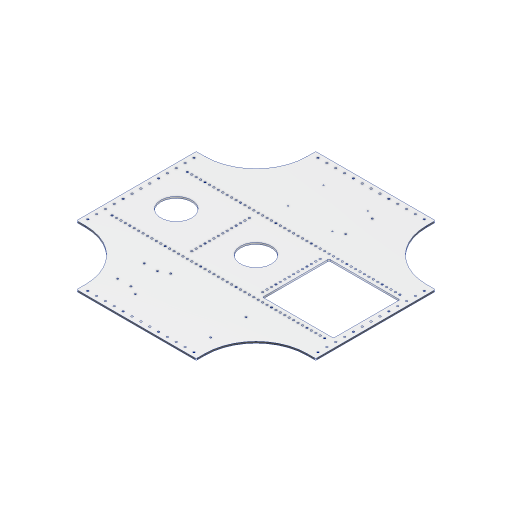
# Autodesk Inventor part: 27in_2_125 belly pan_Green
Saved by Autodesk Inventor 2023 (Build 270158000, 158)
## iProperties
Created: 2023-10-28
Part Number: 27in_2_125 belly pan_Green
Material: Aluminum 6061
Document SubType Name: Modeling
Designer: jackc
Density: 2.7 g/cm^3
Appearance: Aluminum - Flat
Author: jackc
Autodesk Inventor part; units mm, degrees
ref_plane "YZ Plane" through (0, 0, 0) normal (1, 0, 0) x (0, 1, 0)
ref_plane "XZ Plane" through (0, 0, 0) normal (0, 1, 0) x (-1, 0, 0)
ref_plane "XY Plane" through (0, 0, 0) normal (0, 0, 1) x (1, 0, 0)
sketch "Sketch1" plane through (0, 0, 0) normal (0, 1, 0) x (-1, 0, 0)
  line L0 (685.8, 0) -> (685.8, -342.9)
  line L1 (0, 0) -> (0, -342.9)
  line L2 (514.35, -514.35) -> (171.45, -514.35)
  line L3 (514.35, 171.45) -> (171.45, 171.45)
  line L4 (685.8, 0) -> (685.8, 171.45) construction
  line L5 (685.8, 171.45) -> (514.35, 171.45) construction
  line L6 (685.8, -342.9) -> (685.8, -514.35) construction
  line L7 (685.8, -514.35) -> (514.35, -514.35) construction
  line L8 (0, -342.9) -> (0, -514.35) construction
  line L9 (0, -514.35) -> (171.45, -514.35) construction
  line L10 (685.8, 0) -> (660.4, 0)
  line L11 (514.35, 171.45) -> (514.35, 146.05)
  line L12 (171.45, 171.45) -> (171.45, 146.05)
  line L13 (0, 0) -> (25.4, 0)
  line L14 (0, -342.9) -> (25.4, -342.9)
  line L15 (171.45, -514.35) -> (171.45, -488.95)
  line L16 (685.8, -342.9) -> (660.4, -342.9)
  line L17 (514.35, -514.35) -> (514.35, -488.95)
  arc A0 (514.35, 146.05) -> (660.4, 0) centre (660.4, 146.05) ccw
  arc A1 (25.4, 0) -> (171.45, 146.05) centre (25.4, 146.05) ccw
  arc A2 (171.45, -488.95) -> (25.4, -342.9) centre (25.4, -488.95) ccw
  arc A3 (660.4, -342.9) -> (514.35, -488.95) centre (660.4, -488.95) ccw
  dimension "d2" = 685.8
  dimension "d14" = 171.45
  dimension "d15" = 25.4
  dimension "d16" = 25.4
  dimension "d17" = 25.4
  dimension "d18" = 25.4
  dimension "d19" = 25.4
  dimension "d21" = 25.4
  dimension "d22" = 25.4
  constraints: 36 end point, 11 equal length, 8 point on circle, 8 vertical, 6 perpendicular, 4 centre point, 4 horizontal, 2 horizontal alignment, 1 coincident, 1 equal radius
  measures "d2" distance of L6.end L4.end
  measures "d14" distance of L0.start L4.end
  measures "d15" distance of L0.start L10.end
  measures "d16" distance of L1.start L13.end
  measures "d17" distance of L1.end L14.end
  measures "d18" distance of L2.end L15.end
  measures "d19" horizontal distance of A0.centre L4.end
  measures "d21" horizontal distance of L8.end A2.centre
  measures "d22" horizontal distance of A1.centre L8.end
extrude "Extrusion1" add sketch "Sketch1" along normal blind 4.7752
sketch "Sketch2" plane through (0, 0, 0) normal (0, 1, 0) x (1, 0, 0)
  line L0 (-685.8, 342.9) -> (-685.8, 0) projected
  line L1 (-685.8, 50.8) -> (0, 50.8) construction
  line L2 (0, 342.9) -> (0, 0) projected
  line L3 (-0.228, 76.2) -> (-685.8, 76.2) construction
  line L4 (-685.8, 266.7) -> (0, 266.7) construction
  line L5 (0, 292.1) -> (-685.8, 292.1) construction
  line L6 (-685.8, 0) -> (-685.8, 342.9) projected
  arc A0 (-514.35, -146.05) -> (-660.4, 0) centre (-660.4, -146.05) ccw construction
  arc A1 (-660.4, 342.9) -> (-514.35, 488.95) centre (-660.4, 488.95) ccw construction
  line L7 (-660.4, 0) -> (-660.4, 342.9) construction
  line L8 (-469.9, 76.2) -> (-469.9, 266.7) construction
  circle A2 centre (-571.5, 171.45) radius 44.45
  line L9 (-444.5, 76.2) -> (-444.5, 266.7) construction
  line L10 (-342.9, 76.2) -> (-342.9, 266.7) construction
  line L11 (-241.3, 76.2) -> (-241.3, 266.7) construction
  circle A3 centre (-444.5, 88.9) radius 2.8067
  circle A4 centre (-241.3, 88.9) radius 2.8067
  circle A5 centre (-444.5, 114.3) radius 2.8067
  circle A6 centre (-241.3, 114.3) radius 2.8067
  circle A7 centre (-444.5, 139.7) radius 2.8067
  circle A8 centre (-241.3, 139.7) radius 2.8067
  circle A9 centre (-444.5, 165.1) radius 2.8067
  circle A10 centre (-241.3, 165.1) radius 2.8067
  circle A11 centre (-444.5, 190.5) radius 2.8067
  circle A12 centre (-241.3, 190.5) radius 2.8067
  circle A13 centre (-444.5, 215.9) radius 2.8067
  circle A14 centre (-241.3, 215.9) radius 2.8067
  circle A15 centre (-444.5, 241.3) radius 2.8067
  circle A16 centre (-241.3, 241.3) radius 2.8067
  circle A17 centre (-342.9, 171.45) radius 44.45
  line L12 (-228.6, 76.2) -> (-228.6, 266.7)
  line L13 (-25.4, 76.2) -> (-25.4, 266.7)
  line L14 (-228.6, 266.7) -> (-25.4, 266.7)
  line L15 (-25.4, 76.2) -> (-228.6, 76.2)
  circle A18 centre (-444.5, 254) radius 2.8067
  circle A19 centre (-241.3, 254) radius 2.8067
  circle A20 centre (-444.5, 228.6) radius 2.8067
  circle A21 centre (-241.3, 228.6) radius 2.8067
  circle A22 centre (-444.5, 203.2) radius 2.8067
  circle A23 centre (-241.3, 203.2) radius 2.8067
  circle A24 centre (-444.5, 177.8) radius 2.8067
  circle A25 centre (-241.3, 177.8) radius 2.8067
  circle A26 centre (-444.5, 152.4) radius 2.8067
  circle A27 centre (-241.3, 152.4) radius 2.8067
  circle A28 centre (-444.5, 127) radius 2.8067
  circle A29 centre (-241.3, 127) radius 2.8067
  circle A30 centre (-444.5, 101.6) radius 2.8067
  circle A31 centre (-241.3, 101.6) radius 2.8067
  point P0 (-660.4, 171.45)
  dimension "d2" = 685.8
  dimension "d14" = 171.45
  dimension "d15" = 25.4
  dimension "d16" = 25.4
  dimension "d17" = 25.4
  dimension "d18" = 25.4
  dimension "d19" = 25.4
  dimension "d21" = 25.4
  dimension "d22" = 25.4
  dimension "d23" = 25.4
  dimension "d24" = 25.4
  dimension "d25" = 190.5
  dimension "d26" = 50.8
  dimension "d31" = 190.5
  dimension "d47" = 88.9
  dimension "d48" = 88.9
  dimension "d49" = 342.9
  dimension "d50" = 101.6
  dimension "d51" = 101.6
  dimension "d54" = 25.4
  dimension "d61" = 12.7
  dimension "d62" = 25.4
  dimension "d100" = 5.6134
  dimension "d101" = 12.7
  dimension "d102" = 12.7
  dimension "d105" = 25.4
  constraints: 30 centre point, 26 end point, 22 point on line, 6 perpendicular, 4 equal radius, 3 horizontal alignment, 3 midpoint, 3 parallel, 3 vertical, 2 collinear, 1 horizontal, 48 other
  measures "d23" distance between parallel lines of L1 L3
  measures "d24" distance between parallel lines of L5 L4
  measures "d25" distance between parallel lines of L4 L3
  measures "d26" distance of L0.start L5.end
  measures "d31" distance between parallel lines of L8 L7
  measures "d47" diameter of A2
  measures "d48" distance of A2.centre point (-660.4, 171.45)
  measures "d49" distance between parallel lines of L10 L2
  measures "d50" distance between parallel lines of L9 L10
  measures "d51" distance between parallel lines of L11 L10
  measures "d54" distance of A3.centre A5.centre
  measures "d61" distance between parallel lines of L11 L12
  measures "d62" distance between parallel lines of L13 L2
  measures "d100" diameter of A15
  measures "d101" distance of L9.start A3.centre
  measures "d102" distance from line of A18.centre L4
  measures "d105" distance of A18.centre A20.centre
sketch "Sketch3" plane through (0, 0, 0) normal (0, 1, 0) x (1, 0, 0)
  line L0 (-419.1, -98.425) -> (-203.2, -98.425) construction
  line L1 (-203.2, -98.425) -> (-203.2, 3.175) construction
  line L2 (-203.2, 3.175) -> (-419.1, 3.175) construction
  line L3 (-419.1, 3.175) -> (-419.1, -98.425) construction
  line L4 (-482.6, -85.725) -> (-444.5, -85.725) construction
  line L5 (-444.5, -85.725) -> (-444.5, -9.525) construction
  line L6 (-444.5, -9.525) -> (-482.6, -9.525) construction
  line L7 (-482.6, -9.525) -> (-482.6, -85.725) construction
  line L8 (-171.45, -171.45) -> (-514.35, -171.45) construction
  circle A0 centre (-419.1, -98.425) radius 2.4892
  circle A1 centre (-444.5, -85.725) radius 2.4892
  circle A2 centre (-482.6, -85.725) radius 2.4892
  circle A3 centre (-482.6, -9.525) radius 2.4892
  circle A4 centre (-419.1, 3.175) radius 2.4892
  circle A5 centre (-203.2, 3.175) radius 2.4892
  circle A6 centre (-203.2, -98.425) radius 2.4892
  circle A7 centre (-444.5, -9.525) radius 2.4892
  point P0 (0, 0)
  dimension "d63" = 101.6
  dimension "d64" = 215.9
  dimension "d65" = 76.2
  dimension "d66" = 38.1
  dimension "d67" = 73.025
  dimension "d68" = 85.725
  dimension "d69" = 31.75
  dimension "d70" = 25.4
  dimension "d71" = 4.9784
  constraints: 16 end point, 8 centre point, 8 coincident, 7 equal radius, 4 parallel, 2 horizontal, 2 perpendicular
  measures "d63" distance of L2.end L0.start
  measures "d64" distance of L1.end L2.end
  measures "d65" distance of L4.end L5.end
  measures "d66" distance of L5.end L6.end
  measures "d67" distance between parallel lines of L0 L8
  measures "d68" distance between parallel lines of L8 L4
  measures "d69" distance from line of L8.start L1
  measures "d70" distance between parallel lines of L3 L5
  measures "d71" diameter of A4
sketch "Sketch4" plane through (0, 0, 0) normal (0, 1, 0) x (1, 0, 0)
  circle A0 centre (-12.7, 323.85) radius 2.8067
  line L0 (0, 342.9) -> (0, 0) projected
  line L1 (-25.4, 342.9) -> (0, 342.9) projected
  circle A1 centre (-12.7, 298.45) radius 2.8067
  circle A2 centre (-12.7, 273.05) radius 2.8067
  circle A3 centre (-12.7, 247.65) radius 2.8067
  circle A4 centre (-12.7, 222.25) radius 2.8067
  circle A5 centre (-12.7, 196.85) radius 2.8067
  circle A6 centre (-12.7, 171.45) radius 2.8067
  circle A7 centre (-12.7, 146.05) radius 2.8067
  circle A8 centre (-12.7, 120.65) radius 2.8067
  circle A9 centre (-12.7, 95.25) radius 2.8067
  circle A10 centre (-12.7, 69.85) radius 2.8067
  circle A11 centre (-12.7, 44.45) radius 2.8067
  circle A12 centre (-12.7, 19.05) radius 2.8067
  circle A13 centre (-419.1, 501.65) radius 2.8067
  circle A14 centre (-393.7, 501.65) radius 2.8067
  circle A15 centre (-368.3, 501.65) radius 2.8067
  circle A16 centre (-317.5, 501.65) radius 2.8067
  circle A17 centre (-292.1, 501.65) radius 2.8067
  circle A18 centre (-266.7, 501.65) radius 2.8067
  circle A19 centre (-241.3, 501.65) radius 2.8067
  circle A20 centre (-215.9, 501.65) radius 2.8067
  circle A21 centre (-190.5, 501.65) radius 2.8067
  circle A22 centre (-342.9, 501.65) radius 2.8067
  circle A23 centre (-444.5, 501.65) radius 2.8067
  circle A24 centre (-469.9, 501.65) radius 2.8067
  circle A25 centre (-495.3, 501.65) radius 2.8067
  circle A26 centre (-673.1, 95.25) radius 2.8067
  circle A27 centre (-673.1, 120.65) radius 2.8067
  circle A28 centre (-673.1, 146.05) radius 2.8067
  circle A29 centre (-673.1, 196.85) radius 2.8067
  circle A30 centre (-673.1, 222.25) radius 2.8067
  circle A31 centre (-673.1, 247.65) radius 2.8067
  circle A32 centre (-673.1, 273.05) radius 2.8067
  circle A33 centre (-673.1, 298.45) radius 2.8067
  circle A34 centre (-673.1, 323.85) radius 2.8067
  circle A35 centre (-673.1, 171.45) radius 2.8067
  circle A36 centre (-673.1, 69.85) radius 2.8067
  circle A37 centre (-673.1, 44.45) radius 2.8067
  circle A38 centre (-673.1, 19.05) radius 2.8067
  circle A39 centre (-266.7, -158.75) radius 2.8067
  circle A40 centre (-292.1, -158.75) radius 2.8067
  circle A41 centre (-317.5, -158.75) radius 2.8067
  circle A42 centre (-368.3, -158.75) radius 2.8067
  circle A43 centre (-393.7, -158.75) radius 2.8067
  circle A44 centre (-419.1, -158.75) radius 2.8067
  circle A45 centre (-444.5, -158.75) radius 2.8067
  circle A46 centre (-469.9, -158.75) radius 2.8067
  circle A47 centre (-495.3, -158.75) radius 2.8067
  circle A48 centre (-342.9, -158.75) radius 2.8067
  circle A49 centre (-241.3, -158.75) radius 2.8067
  circle A50 centre (-215.9, -158.75) radius 2.8067
  circle A51 centre (-190.5, -158.75) radius 2.8067
  circle A52 centre (-38.1, 279.4) radius 2.8067
  line L2 (-228.6, 266.7) -> (-25.4, 266.7)
  line L3 (-228.6, 171.45) -> (-25.4, 171.45) construction
  line L4 (-514.35, 514.35) -> (-171.45, 514.35) construction
  line L5 (-241.3, 171.45) -> (-38.1, 171.45) construction
  circle A53 centre (-50.8, 279.4) radius 2.8067
  line L6 (-254, 171.45) -> (-50.8, 171.45) construction
  circle A54 centre (-63.5, 279.4) radius 2.8067
  line L7 (-266.7, 171.45) -> (-63.5, 171.45) construction
  circle A55 centre (-76.2, 279.4) radius 2.8067
  line L8 (-279.4, 171.45) -> (-76.2, 171.45) construction
  circle A56 centre (-88.9, 279.4) radius 2.8067
  line L9 (-292.1, 171.45) -> (-88.9, 171.45) construction
  circle A57 centre (-101.6, 279.4) radius 2.8067
  line L10 (-304.8, 171.45) -> (-101.6, 171.45) construction
  circle A58 centre (-114.3, 279.4) radius 2.8067
  line L11 (-317.5, 171.45) -> (-114.3, 171.45) construction
  circle A59 centre (-127, 279.4) radius 2.8067
  line L12 (-330.2, 171.45) -> (-127, 171.45) construction
  circle A60 centre (-139.7, 279.4) radius 2.8067
  line L13 (-342.9, 171.45) -> (-139.7, 171.45) construction
  circle A61 centre (-152.4, 279.4) radius 2.8067
  line L14 (-355.6, 171.45) -> (-152.4, 171.45) construction
  circle A62 centre (-165.1, 279.4) radius 2.8067
  line L15 (-368.3, 171.45) -> (-165.1, 171.45) construction
  circle A63 centre (-177.8, 279.4) radius 2.8067
  line L16 (-381, 171.45) -> (-177.8, 171.45) construction
  circle A64 centre (-190.5, 279.4) radius 2.8067
  line L17 (-393.7, 171.45) -> (-190.5, 171.45) construction
  circle A65 centre (-203.2, 279.4) radius 2.8067
  line L18 (-406.4, 171.45) -> (-203.2, 171.45) construction
  circle A66 centre (-215.9, 279.4) radius 2.8067
  line L19 (-419.1, 171.45) -> (-215.9, 171.45) construction
  circle A67 centre (-228.6, 279.4) radius 2.8067
  line L20 (-431.8, 171.45) -> (-228.6, 171.45) construction
  circle A68 centre (-241.3, 279.4) radius 2.8067
  line L21 (-444.5, 171.45) -> (-241.3, 171.45) construction
  circle A69 centre (-254, 279.4) radius 2.8067
  line L22 (-457.2, 171.45) -> (-254, 171.45) construction
  circle A70 centre (-266.7, 279.4) radius 2.8067
  line L23 (-469.9, 171.45) -> (-266.7, 171.45) construction
  circle A71 centre (-279.4, 279.4) radius 2.8067
  line L24 (-482.6, 171.45) -> (-279.4, 171.45) construction
  circle A72 centre (-292.1, 279.4) radius 2.8067
  line L25 (-495.3, 171.45) -> (-292.1, 171.45) construction
  circle A73 centre (-304.8, 279.4) radius 2.8067
  line L26 (-508, 171.45) -> (-304.8, 171.45) construction
  circle A74 centre (-317.5, 279.4) radius 2.8067
  line L27 (-520.7, 171.45) -> (-317.5, 171.45) construction
  circle A75 centre (-330.2, 279.4) radius 2.8067
  line L28 (-533.4, 171.45) -> (-330.2, 171.45) construction
  circle A76 centre (-342.9, 279.4) radius 2.8067
  line L29 (-546.1, 171.45) -> (-342.9, 171.45) construction
  circle A77 centre (-355.6, 279.4) radius 2.8067
  line L30 (-558.8, 171.45) -> (-355.6, 171.45) construction
  circle A78 centre (-368.3, 279.4) radius 2.8067
  line L31 (-571.5, 171.45) -> (-368.3, 171.45) construction
  circle A79 centre (-381, 279.4) radius 2.8067
  line L32 (-584.2, 171.45) -> (-381, 171.45) construction
  circle A80 centre (-393.7, 279.4) radius 2.8067
  line L33 (-596.9, 171.45) -> (-393.7, 171.45) construction
  circle A81 centre (-406.4, 279.4) radius 2.8067
  line L34 (-609.6, 171.45) -> (-406.4, 171.45) construction
  circle A82 centre (-419.1, 279.4) radius 2.8067
  line L35 (-622.3, 171.45) -> (-419.1, 171.45) construction
  circle A83 centre (-431.8, 279.4) radius 2.8067
  line L36 (-635, 171.45) -> (-431.8, 171.45) construction
  circle A84 centre (-444.5, 279.4) radius 2.8067
  line L37 (-647.7, 171.45) -> (-444.5, 171.45) construction
  circle A85 centre (-457.2, 279.4) radius 2.8067
  line L38 (-660.4, 171.45) -> (-457.2, 171.45) construction
  circle A86 centre (-469.9, 279.4) radius 2.8067
  line L39 (-673.1, 171.45) -> (-469.9, 171.45) construction
  circle A87 centre (-482.6, 279.4) radius 2.8067
  line L40 (-685.8, 171.45) -> (-482.6, 171.45) construction
  circle A88 centre (-495.3, 279.4) radius 2.8067
  line L41 (-698.5, 171.45) -> (-495.3, 171.45) construction
  circle A89 centre (-508, 279.4) radius 2.8067
  line L42 (-711.2, 171.45) -> (-508, 171.45) construction
  circle A90 centre (-520.7, 279.4) radius 2.8067
  line L43 (-723.9, 171.45) -> (-520.7, 171.45) construction
  circle A91 centre (-533.4, 279.4) radius 2.8067
  line L44 (-736.6, 171.45) -> (-533.4, 171.45) construction
  circle A92 centre (-546.1, 279.4) radius 2.8067
  line L45 (-749.3, 171.45) -> (-546.1, 171.45) construction
  circle A93 centre (-558.8, 279.4) radius 2.8067
  line L46 (-762, 171.45) -> (-558.8, 171.45) construction
  circle A94 centre (-571.5, 279.4) radius 2.8067
  line L47 (-774.7, 171.45) -> (-571.5, 171.45) construction
  circle A95 centre (-584.2, 279.4) radius 2.8067
  line L48 (-787.4, 171.45) -> (-584.2, 171.45) construction
  circle A96 centre (-596.9, 279.4) radius 2.8067
  line L49 (-800.1, 171.45) -> (-596.9, 171.45) construction
  circle A97 centre (-609.6, 279.4) radius 2.8067
  line L50 (-812.8, 171.45) -> (-609.6, 171.45) construction
  circle A98 centre (-622.3, 279.4) radius 2.8067
  line L51 (-825.5, 171.45) -> (-622.3, 171.45) construction
  circle A99 centre (-635, 279.4) radius 2.8067
  line L52 (-838.2, 171.45) -> (-635, 171.45) construction
  circle A100 centre (-647.7, 279.4) radius 2.8067
  circle A101 centre (-38.1, 63.5) radius 2.8067
  circle A102 centre (-50.8, 63.5) radius 2.8067
  circle A103 centre (-63.5, 63.5) radius 2.8067
  circle A104 centre (-76.2, 63.5) radius 2.8067
  circle A105 centre (-88.9, 63.5) radius 2.8067
  circle A106 centre (-101.6, 63.5) radius 2.8067
  circle A107 centre (-114.3, 63.5) radius 2.8067
  circle A108 centre (-127, 63.5) radius 2.8067
  circle A109 centre (-139.7, 63.5) radius 2.8067
  circle A110 centre (-152.4, 63.5) radius 2.8067
  circle A111 centre (-165.1, 63.5) radius 2.8067
  circle A112 centre (-177.8, 63.5) radius 2.8067
  circle A113 centre (-190.5, 63.5) radius 2.8067
  circle A114 centre (-203.2, 63.5) radius 2.8067
  circle A115 centre (-215.9, 63.5) radius 2.8067
  circle A116 centre (-228.6, 63.5) radius 2.8067
  circle A117 centre (-241.3, 63.5) radius 2.8067
  circle A118 centre (-254, 63.5) radius 2.8067
  circle A119 centre (-266.7, 63.5) radius 2.8067
  circle A120 centre (-279.4, 63.5) radius 2.8067
  circle A121 centre (-292.1, 63.5) radius 2.8067
  circle A122 centre (-304.8, 63.5) radius 2.8067
  circle A123 centre (-317.5, 63.5) radius 2.8067
  circle A124 centre (-330.2, 63.5) radius 2.8067
  circle A125 centre (-342.9, 63.5) radius 2.8067
  circle A126 centre (-355.6, 63.5) radius 2.8067
  circle A127 centre (-368.3, 63.5) radius 2.8067
  circle A128 centre (-381, 63.5) radius 2.8067
  circle A129 centre (-393.7, 63.5) radius 2.8067
  circle A130 centre (-406.4, 63.5) radius 2.8067
  circle A131 centre (-419.1, 63.5) radius 2.8067
  circle A132 centre (-431.8, 63.5) radius 2.8067
  circle A133 centre (-444.5, 63.5) radius 2.8067
  circle A134 centre (-457.2, 63.5) radius 2.8067
  circle A135 centre (-469.9, 63.5) radius 2.8067
  circle A136 centre (-482.6, 63.5) radius 2.8067
  circle A137 centre (-495.3, 63.5) radius 2.8067
  circle A138 centre (-508, 63.5) radius 2.8067
  circle A139 centre (-520.7, 63.5) radius 2.8067
  circle A140 centre (-533.4, 63.5) radius 2.8067
  circle A141 centre (-546.1, 63.5) radius 2.8067
  circle A142 centre (-558.8, 63.5) radius 2.8067
  circle A143 centre (-571.5, 63.5) radius 2.8067
  circle A144 centre (-584.2, 63.5) radius 2.8067
  circle A145 centre (-596.9, 63.5) radius 2.8067
  circle A146 centre (-609.6, 63.5) radius 2.8067
  circle A147 centre (-622.3, 63.5) radius 2.8067
  circle A148 centre (-635, 63.5) radius 2.8067
  circle A149 centre (-647.7, 63.5) radius 2.8067
  point P0 (-12.7, 342.9)
  point P1 (-342.9, 171.45)
  dimension "d2" = 685.8
  dimension "d14" = 171.45
  dimension "d15" = 25.4
  dimension "d16" = 25.4
  dimension "d17" = 25.4
  dimension "d18" = 25.4
  dimension "d19" = 25.4
  dimension "d21" = 25.4
  dimension "d22" = 25.4
  dimension "d74" = 12.7
  dimension "d75" = 5.6134
  dimension "d76" = 19.05
  dimension "d79" = 25.4
  dimension "d86" = 360
  dimension "d88" = 12.7
  dimension "d89" = 12.7
  dimension "d90" = 342.9
  dimension "d93" = 12.7
  constraints: 150 centre point, 100 end point, 49 symmetric about line, 1 equal radius, 1 horizontal, 1 midpoint, 1 vertical, 418 other
  measures "d74" distance from line of L0 A0.centre
  measures "d75" diameter of A0
  measures "d76" distance of A0.centre point (-12.7, 342.9)
  measures "d79" distance of A0.centre A1.centre
  measures "d88" horizontal distance of A52.centre L2.end
  measures "d89" horizontal distance of L2.end A52.centre
  measures "d90" distance between parallel lines of L3 L4
  measures "d93" distance of L3.start L5.start
sketch "Sketch6" plane through (0, 0, 0) normal (0, 1, 0) x (1, 0, 0)
  line L0 (-171.45, -146.05) -> (-171.45, -171.45) projected
  arc A0 (-25.4, 0) -> (-171.45, -146.05) centre (-25.4, -146.05) ccw projected
  line L1 (0, 0) -> (-25.4, 0) projected
  line L2 (0, 342.9) -> (0, 0) projected
  line L3 (-25.4, 342.9) -> (0, 342.9) projected
  arc A1 (-171.45, 488.95) -> (-25.4, 342.9) centre (-25.4, 488.95) ccw projected
  line L4 (-171.45, 514.35) -> (-171.45, 488.95) projected
  line L5 (-514.35, 514.35) -> (-171.45, 514.35) projected
  line L6 (-514.35, 488.95) -> (-514.35, 514.35) projected
  arc A2 (-660.4, 342.9) -> (-514.35, 488.95) centre (-660.4, 488.95) ccw projected
  line L7 (-685.8, 342.9) -> (-660.4, 342.9) projected
  line L8 (-685.8, 0) -> (-685.8, 342.9) projected
  line L9 (-660.4, 0) -> (-685.8, 0) projected
  arc A3 (-514.35, -146.05) -> (-660.4, 0) centre (-660.4, -146.05) ccw projected
  line L10 (-514.35, -171.45) -> (-514.35, -146.05) projected
  line L11 (-171.45, -171.45) -> (-514.35, -171.45) projected
  line L12 (-419.1, 441.325) -> (-292.1, 441.325) construction
  line L13 (-292.1, 441.325) -> (-292.1, 339.725) construction
  line L14 (-292.1, 339.725) -> (-419.1, 339.725) construction
  line L15 (-419.1, 339.725) -> (-419.1, 441.325) construction
  circle A4 centre (-419.1, 441.325) radius 1.651
  circle A5 centre (-292.1, 441.325) radius 1.651
  circle A6 centre (-292.1, 339.725) radius 1.651
  circle A7 centre (-419.1, 339.725) radius 1.651
  circle A8 centre (-266.7, 428.625) radius 2.54
  circle A9 centre (-266.7, 352.425) radius 2.54
  dimension "d2" = 685.8
  dimension "d14" = 171.45
  dimension "d15" = 25.4
  dimension "d16" = 25.4
  dimension "d17" = 25.4
  dimension "d18" = 25.4
  dimension "d19" = 25.4
  dimension "d21" = 25.4
  dimension "d22" = 25.4
  dimension "d110" = 127
  dimension "d111" = 101.6
  dimension "d112" = 3.302
  dimension "d115" = 76.2
  dimension "d116" = 25.4
  dimension "d117" = 12.7
  dimension "d118" = 5.08
  dimension "d124" = 266.7
  constraints: 8 end point, 6 centre point, 4 coincident, 4 equal radius, 2 parallel, 1 horizontal, 1 perpendicular, 1 vertical alignment
  measures "d110" distance of L12.start L12.end
  measures "d111" distance of L14.end L12.start
  measures "d112" diameter of A4
  measures "d115" distance of A9.centre A8.centre
  measures "d116" horizontal distance of A8.centre L12.end
  measures "d117" vertical distance of A9.centre L13.end
  measures "d118" diameter of A9
  measures "d124" distance from line of L15 L7.start
hole "Hole1" at (-203.2, 0, 98.425) at (-203.2, 0, -3.175) at (-419.1, 0, -3.175) at (-419.1, 0, 98.425) at (-444.5, 0, 85.725) at (-444.5, 0, 9.525) at (-482.6, 0, 9.525) at (-482.6, 0, 85.725) direction (0, 1, 0) diameter 4.9784 end through all countersink diameter 9.525 countersink angle 82
hole "Hole2" at (-266.7, 0, -428.625) at (-266.7, 0, -352.425) direction (0, 1, 0) diameter 4.9784 end through all countersink diameter 9.525 countersink angle 82
extrude "Extrusion6" cut sketch "Sketch2" along normal blind 6.35
extrude "Extrusion7" cut sketch "Sketch4" along normal blind 6.35
sketch "Sketch8" plane through (0, 0, 0) normal (0, -1, 0) x (1, 0, 0)
  circle A0 centre (-622.3, -63.5) radius 2.8067 projected
  circle A1 centre (-571.5, -63.5) radius 2.8067 projected
  circle A2 centre (-520.7, -63.5) radius 2.8067 projected
  circle A3 centre (-469.9, -63.5) radius 2.8067 projected
  circle A4 centre (-419.1, -63.5) radius 2.8067 projected
  circle A5 centre (-355.6, -63.5) radius 2.8067 projected
  circle A6 centre (-317.5, -63.5) radius 2.8067 projected
  circle A7 centre (-266.7, -63.5) radius 2.8067 projected
  circle A8 centre (-215.9, -63.5) radius 2.8067 projected
  circle A9 centre (-165.1, -63.5) radius 2.8067 projected
  circle A10 centre (-63.5, -63.5) radius 2.8067 projected
  circle A11 centre (-114.3, -63.5) radius 2.8067 projected
  circle A12 centre (-50.8, -279.4) radius 2.8067 projected
  circle A13 centre (-101.6, -279.4) radius 2.8067 projected
  circle A14 centre (-152.4, -279.4) radius 2.8067 projected
  circle A15 centre (-203.2, -279.4) radius 2.8067 projected
  circle A16 centre (-254, -279.4) radius 2.8067 projected
  circle A17 centre (-304.8, -279.4) radius 2.8067 projected
  circle A18 centre (-355.6, -279.4) radius 2.8067 projected
  circle A19 centre (-406.4, -279.4) radius 2.8067 projected
  circle A20 centre (-457.2, -279.4) radius 2.8067 projected
  circle A21 centre (-508, -279.4) radius 2.8067 projected
  circle A22 centre (-558.8, -279.4) radius 2.8067 projected
  circle A23 centre (-609.6, -279.4) radius 2.8067 projected
  circle A24 centre (-190.5, -501.65) radius 2.8067 projected
  circle A25 centre (-292.1, -501.65) radius 2.8067 projected
  circle A26 centre (-393.7, -501.65) radius 2.8067 projected
  circle A27 centre (-495.3, -501.65) radius 2.8067 projected
  circle A28 centre (-673.1, -247.65) radius 2.8067 projected
  circle A29 centre (-673.1, -146.05) radius 2.8067 projected
  circle A30 centre (-673.1, -19.05) radius 2.8067 projected
  circle A31 centre (-241.3, 158.75) radius 2.8067 projected
  circle A32 centre (-342.9, 158.75) radius 2.8067 projected
  circle A33 centre (-444.5, 158.75) radius 2.8067 projected
  circle A34 centre (-12.7, -44.45) radius 2.8067 projected
  circle A35 centre (-12.7, -146.05) radius 2.8067 projected
  circle A36 centre (-12.7, -247.65) radius 2.8067 projected
  circle A37 centre (-12.7, -323.85) radius 2.8067 projected
  circle A38 centre (-12.7, -222.25) radius 2.8067 projected
  circle A39 centre (-12.7, -120.65) radius 2.8067 projected
  circle A40 centre (-12.7, -19.05) radius 2.8067 projected
  circle A41 centre (-419.1, 158.75) radius 2.8067 projected
  circle A42 centre (-317.5, 158.75) radius 2.8067 projected
  circle A43 centre (-215.9, 158.75) radius 2.8067 projected
  circle A44 centre (-673.1, -69.85) radius 2.8067 projected
  circle A45 centre (-673.1, -171.45) radius 2.8067 projected
  circle A46 centre (-673.1, -273.05) radius 2.8067 projected
  circle A47 centre (-469.9, -501.65) radius 2.8067 projected
  circle A48 centre (-368.3, -501.65) radius 2.8067 projected
  circle A49 centre (-266.7, -501.65) radius 2.8067 projected
  circle A50 centre (-622.3, -279.4) radius 2.8067 projected
  circle A51 centre (-596.9, -279.4) radius 2.8067 projected
  circle A52 centre (-546.1, -279.4) radius 2.8067 projected
  circle A53 centre (-495.3, -279.4) radius 2.8067 projected
  circle A54 centre (-444.5, -279.4) radius 2.8067 projected
  circle A55 centre (-393.7, -279.4) radius 2.8067 projected
  circle A56 centre (-342.9, -279.4) radius 2.8067 projected
  circle A57 centre (-292.1, -279.4) radius 2.8067 projected
  circle A58 centre (-241.3, -279.4) radius 2.8067 projected
  circle A59 centre (-177.8, -279.4) radius 2.8067 projected
  circle A60 centre (-139.7, -279.4) radius 2.8067 projected
  circle A61 centre (-88.9, -279.4) radius 2.8067 projected
  circle A62 centre (-38.1, -279.4) radius 2.8067 projected
  circle A63 centre (-101.6, -63.5) radius 2.8067 projected
  circle A64 centre (-50.8, -63.5) radius 2.8067 projected
  circle A65 centre (-177.8, -63.5) radius 2.8067 projected
  circle A66 centre (-228.6, -63.5) radius 2.8067 projected
  circle A67 centre (-279.4, -63.5) radius 2.8067 projected
  circle A68 centre (-330.2, -63.5) radius 2.8067 projected
  circle A69 centre (-381, -63.5) radius 2.8067 projected
  circle A70 centre (-431.8, -63.5) radius 2.8067 projected
  circle A71 centre (-482.6, -63.5) radius 2.8067 projected
  circle A72 centre (-533.4, -63.5) radius 2.8067 projected
  circle A73 centre (-584.2, -63.5) radius 2.8067 projected
  circle A74 centre (-635, -63.5) radius 2.8067 projected
  circle A75 centre (-609.6, -63.5) radius 2.8067 projected
  circle A76 centre (-558.8, -63.5) radius 2.8067 projected
  circle A77 centre (-508, -63.5) radius 2.8067 projected
  circle A78 centre (-457.2, -63.5) radius 2.8067 projected
  circle A79 centre (-406.4, -63.5) radius 2.8067 projected
  circle A80 centre (-368.3, -63.5) radius 2.8067 projected
  circle A81 centre (-304.8, -63.5) radius 2.8067 projected
  circle A82 centre (-254, -63.5) radius 2.8067 projected
  circle A83 centre (-203.2, -63.5) radius 2.8067 projected
  circle A84 centre (-152.4, -63.5) radius 2.8067 projected
  circle A85 centre (-76.2, -63.5) radius 2.8067 projected
  circle A86 centre (-127, -63.5) radius 2.8067 projected
  circle A87 centre (-63.5, -279.4) radius 2.8067 projected
  circle A88 centre (-114.3, -279.4) radius 2.8067 projected
  circle A89 centre (-165.1, -279.4) radius 2.8067 projected
  circle A90 centre (-215.9, -279.4) radius 2.8067 projected
  circle A91 centre (-266.7, -279.4) radius 2.8067 projected
  circle A92 centre (-317.5, -279.4) radius 2.8067 projected
  circle A93 centre (-368.3, -279.4) radius 2.8067 projected
  circle A94 centre (-419.1, -279.4) radius 2.8067 projected
  circle A95 centre (-469.9, -279.4) radius 2.8067 projected
  circle A96 centre (-520.7, -279.4) radius 2.8067 projected
  circle A97 centre (-571.5, -279.4) radius 2.8067 projected
  circle A98 centre (-635, -279.4) radius 2.8067 projected
  circle A99 centre (-215.9, -501.65) radius 2.8067 projected
  circle A100 centre (-317.5, -501.65) radius 2.8067 projected
  circle A101 centre (-419.1, -501.65) radius 2.8067 projected
  circle A102 centre (-673.1, -323.85) radius 2.8067 projected
  circle A103 centre (-673.1, -222.25) radius 2.8067 projected
  circle A104 centre (-673.1, -120.65) radius 2.8067 projected
  circle A105 centre (-673.1, -44.45) radius 2.8067 projected
  circle A106 centre (-266.7, 158.75) radius 2.8067 projected
  circle A107 centre (-368.3, 158.75) radius 2.8067 projected
  circle A108 centre (-469.9, 158.75) radius 2.8067 projected
  circle A109 centre (-12.7, -69.85) radius 2.8067 projected
  circle A110 centre (-12.7, -171.45) radius 2.8067 projected
  circle A111 centre (-12.7, -273.05) radius 2.8067 projected
  circle A112 centre (-12.7, -298.45) radius 2.8067 projected
  circle A113 centre (-12.7, -196.85) radius 2.8067 projected
  circle A114 centre (-12.7, -95.25) radius 2.8067 projected
  circle A115 centre (-495.3, 158.75) radius 2.8067 projected
  circle A116 centre (-393.7, 158.75) radius 2.8067 projected
  circle A117 centre (-292.1, 158.75) radius 2.8067 projected
  circle A118 centre (-190.5, 158.75) radius 2.8067 projected
  circle A119 centre (-673.1, -95.25) radius 2.8067 projected
  circle A120 centre (-673.1, -196.85) radius 2.8067 projected
  circle A121 centre (-673.1, -298.45) radius 2.8067 projected
  circle A122 centre (-444.5, -501.65) radius 2.8067 projected
  circle A123 centre (-342.9, -501.65) radius 2.8067 projected
  circle A124 centre (-241.3, -501.65) radius 2.8067 projected
  circle A125 centre (-647.7, -279.4) radius 2.8067 projected
  circle A126 centre (-584.2, -279.4) radius 2.8067 projected
  circle A127 centre (-533.4, -279.4) radius 2.8067 projected
  circle A128 centre (-482.6, -279.4) radius 2.8067 projected
  circle A129 centre (-431.8, -279.4) radius 2.8067 projected
  circle A130 centre (-381, -279.4) radius 2.8067 projected
  circle A131 centre (-330.2, -279.4) radius 2.8067 projected
  circle A132 centre (-279.4, -279.4) radius 2.8067 projected
  circle A133 centre (-228.6, -279.4) radius 2.8067 projected
  circle A134 centre (-190.5, -279.4) radius 2.8067 projected
  circle A135 centre (-127, -279.4) radius 2.8067 projected
  circle A136 centre (-76.2, -279.4) radius 2.8067 projected
  circle A137 centre (-139.7, -63.5) radius 2.8067 projected
  circle A138 centre (-88.9, -63.5) radius 2.8067 projected
  circle A139 centre (-38.1, -63.5) radius 2.8067 projected
  circle A140 centre (-190.5, -63.5) radius 2.8067 projected
  circle A141 centre (-241.3, -63.5) radius 2.8067 projected
  circle A142 centre (-292.1, -63.5) radius 2.8067 projected
  circle A143 centre (-342.9, -63.5) radius 2.8067 projected
  circle A144 centre (-393.7, -63.5) radius 2.8067 projected
  circle A145 centre (-444.5, -63.5) radius 2.8067 projected
  circle A146 centre (-495.3, -63.5) radius 2.8067 projected
  circle A147 centre (-546.1, -63.5) radius 2.8067 projected
  circle A148 centre (-596.9, -63.5) radius 2.8067 projected
  circle A149 centre (-647.7, -63.5) radius 2.8067 projected
  circle A150 centre (-241.3, -114.3) radius 2.8067 projected
  circle A151 centre (-241.3, -165.1) radius 2.8067 projected
  circle A152 centre (-241.3, -215.9) radius 2.8067 projected
  circle A153 centre (-444.5, -254) radius 2.8067 projected
  circle A154 centre (-444.5, -203.2) radius 2.8067 projected
  circle A155 centre (-444.5, -152.4) radius 2.8067 projected
  circle A156 centre (-444.5, -101.6) radius 2.8067 projected
  circle A157 centre (-571.5, -171.45) radius 44.45 projected
  circle A158 centre (-444.5, -88.9) radius 2.8067 projected
  circle A159 centre (-444.5, -139.7) radius 2.8067 projected
  circle A160 centre (-444.5, -190.5) radius 2.8067 projected
  circle A161 centre (-444.5, -241.3) radius 2.8067 projected
  circle A162 centre (-241.3, -228.6) radius 2.8067 projected
  circle A163 centre (-241.3, -177.8) radius 2.8067 projected
  circle A164 centre (-241.3, -127) radius 2.8067 projected
  circle A165 centre (-241.3, -101.6) radius 2.8067 projected
  circle A166 centre (-241.3, -152.4) radius 2.8067 projected
  circle A167 centre (-241.3, -203.2) radius 2.8067 projected
  circle A168 centre (-241.3, -254) radius 2.8067 projected
  circle A169 centre (-444.5, -215.9) radius 2.8067 projected
  circle A170 centre (-444.5, -165.1) radius 2.8067 projected
  circle A171 centre (-444.5, -114.3) radius 2.8067 projected
  circle A172 centre (-342.9, -171.45) radius 44.45 projected
  line L0 (-25.4, -76.2) -> (-25.4, -266.7) projected
  line L1 (-25.4, -266.7) -> (-228.6, -266.7) projected
  line L2 (-228.6, -266.7) -> (-228.6, -76.2) projected
  line L3 (-228.6, -76.2) -> (-25.4, -76.2) projected
  circle A173 centre (-444.5, -127) radius 2.8067 projected
  circle A174 centre (-444.5, -177.8) radius 2.8067 projected
  circle A175 centre (-444.5, -228.6) radius 2.8067 projected
  circle A176 centre (-241.3, -241.3) radius 2.8067 projected
  circle A177 centre (-241.3, -190.5) radius 2.8067 projected
  circle A178 centre (-241.3, -139.7) radius 2.8067 projected
  circle A179 centre (-241.3, -88.9) radius 2.8067 projected
  circle A180 centre (-266.7, -428.625) radius 4.7625 projected
  circle A181 centre (-266.7, -352.425) radius 4.7625 projected
  circle A182 centre (-482.6, 9.525) radius 4.7625 projected
  circle A183 centre (-444.5, 85.725) radius 4.7625 projected
  circle A184 centre (-419.1, -3.175) radius 4.7625 projected
  circle A185 centre (-203.2, 98.425) radius 4.7625 projected
  circle A186 centre (-203.2, -3.175) radius 4.7625 projected
  circle A187 centre (-419.1, 98.425) radius 4.7625 projected
  circle A188 centre (-444.5, 9.525) radius 4.7625 projected
  circle A189 centre (-482.6, 85.725) radius 4.7625 projected
  line L4 (-514.35, 171.45) -> (-171.45, 171.45) projected
  line L5 (-514.35, 146.05) -> (-514.35, 171.45) projected
  arc A190 (-660.4, 0) -> (-514.35, 146.05) centre (-660.4, 146.05) ccw projected
  line L6 (-685.8, 0) -> (-660.4, 0) projected
  line L7 (-685.8, -342.9) -> (-685.8, 0) projected
  line L8 (-660.4, -342.9) -> (-685.8, -342.9) projected
  arc A191 (-514.35, -488.95) -> (-660.4, -342.9) centre (-660.4, -488.95) ccw projected
  line L9 (-514.35, -514.35) -> (-514.35, -488.95) projected
  line L10 (-171.45, -514.35) -> (-514.35, -514.35) projected
  line L11 (-171.45, -488.95) -> (-171.45, -514.35) projected
  arc A192 (-25.4, -342.9) -> (-171.45, -488.95) centre (-25.4, -488.95) ccw projected
  line L12 (0, -342.9) -> (-25.4, -342.9) projected
  line L13 (0, 0) -> (0, -342.9) projected
  line L14 (-25.4, 0) -> (0, 0) projected
  arc A193 (-171.45, 146.05) -> (-25.4, 0) centre (-25.4, 146.05) ccw projected
  line L15 (-171.45, 171.45) -> (-171.45, 146.05) projected
  dimension "d2" = 685.8
  dimension "d14" = 171.45
  dimension "d15" = 25.4
  dimension "d16" = 25.4
  dimension "d17" = 25.4
  dimension "d18" = 25.4
  dimension "d19" = 25.4
  dimension "d21" = 25.4
  dimension "d22" = 25.4
hole "Hole5" at (-12.7, 0, -19.05) at (-12.7, 0, -120.65) at (-12.7, 0, -222.25) at (-12.7, 0, -323.85) at (-38.1, 0, -63.5) at (-38.1, 0, -279.4) at (-88.9, 0, -63.5) at (-88.9, 0, -279.4) at (-241.3, 0, -127) at (-241.3, 0, -215.9) at (-292.1, 0, -63.5) at (-292.1, 0, -279.4) at (-393.7, 0, -63.5) at (-393.7, 0, -279.4) at (-444.5, 0, -127) at (-444.5, 0, -215.9) at (-495.3, 0, -63.5) at (-495.3, 0, -279.4) at (-647.7, 0, -279.4) at (-647.7, 0, -63.5) at (-596.9, 0, -63.5) at (-596.9, 0, -279.4) at (-673.1, 0, -323.85) at (-673.1, 0, -222.25) at (-673.1, 0, -120.65) at (-673.1, 0, -19.05) at (-190.5, 0, -63.5) at (-190.5, 0, -279.4) at (-190.5, 0, -501.65) at (-292.1, 0, -501.65) at (-495.3, 0, -501.65) at (-393.7, 0, -501.65) at (-190.5, 0, 158.75) at (-495.3, 0, 158.75) at (-292.1, 0, 158.75) at (-393.7, 0, 158.75) direction (0, 1, 0) diameter 5.6134 end through all countersink diameter 11.1125 countersink angle 82
fillet "Fillet2" radius 3.175 4 edges at (-228.6, 2.3876, -266.7) (-25.4, 2.3876, -266.7) (-228.6, 2.3876, -76.2) (-25.4, 2.3876, -76.2)
fillet "Fillet3" radius 3.175 8 edges at (-171.45, 2.3876, 171.45) (0, 2.3876, 0) (0, 2.3876, -342.9) (-171.45, 2.3876, -514.35) (-514.35, 2.3876, -514.35) (-685.8, 2.3876, -342.9) (-685.8, 2.3876, 0) (-514.35, 2.3876, 171.45)
hole "Hole6" at (-292.1, 0, -441.325) at (-292.1, 0, -339.725) at (-419.1, 0, -339.725) at (-419.1, 0, -441.325) direction (0, 1, 0) diameter 3.2766 end through all countersink diameter 7.1628 countersink angle 82
equation "\"d21\" = d22"
equation "\"d22\" = d19"
equation "\"d51\" = d50"
body "Solid1"
